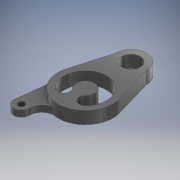
# Autodesk Inventor part: LR3_2
Saved by Autodesk Inventor 2018 (Build 220112000, 112)
## iProperties
Created: 2020-04-08
Part Number: LR3_2
Material: Типовые
Document SubType Name: Modeling
Designer: Siarhei
Density: 1 g/cm^3
Appearance: По умолчанию
Author: Siarhei
Autodesk Inventor part; units mm, degrees
ref_plane "YZ Plane" through (0, 0, 0) normal (1, 0, 0) x (0, 1, 0)
ref_plane "XZ Plane" through (0, 0, 0) normal (0, 1, 0) x (-1, 0, 0)
ref_plane "XY Plane" through (0, 0, 0) normal (0, 0, 1) x (1, 0, 0)
sketch "Эскиз1" plane through (0, 0, 0) normal (0, 0, 1) x (1, 0, 0)
  circle A0 centre (0, 0) radius 5
  circle A1 centre (0, 0) radius 12.5
  arc A2 (-2.4853, 79.8323) -> (82.4853, 79.8323) centre (40, 65) ccw
  arc A3 (57.6777, 47.3223) -> (22.3223, 47.3223) centre (40, 65) ccw construction
  arc A4 (64.7487, 40.2513) -> (15.2513, 40.2513) centre (40, 65) ccw
  arc A5 (50.6066, 54.3934) -> (29.3934, 54.3934) centre (40, 65) ccw
  arc A6 (50.6066, 54.3934) -> (64.7487, 40.2513) centre (57.6777, 47.3223) ccw
  arc A7 (15.2513, 40.2513) -> (29.3934, 54.3934) centre (22.3223, 47.3223) ccw
  line L0 (40, 65) -> (57.6777, 47.3223) construction
  line L1 (40, 65) -> (65, 65) construction
  line L2 (40, 65) -> (22.3223, 47.3223) construction
  line L3 (-12.5, 0) -> (-5, 65)
  circle A8 centre (40, 140) radius 15
  arc A9 (65, 140) -> (15, 140) centre (40, 140) ccw
  line L4 (15, 140) -> (-3.8175, 75.2482)
  line L5 (65, 140) -> (83.8175, 75.2482)
  arc A10 (31.1612, 20.8766) -> (12.5, 0) centre (32.4788, 0.92) ccw
  dimension "d0" = 10
  dimension "d1" = 25
  dimension "d2" = 90
  dimension "d4" = 25
  dimension "d5" = 45
  dimension "d6" = 90
  dimension "d7" = 20
  dimension "d9" = 30
  dimension "d10" = 50
  dimension "d11" = 20
  dimension "d24" = 73.796
  dimension "d25" = 32.409
  dimension "d26" = 22.786
  dimension "d27" = 101.4868
  dimension "d28" = 65
  dimension "d29" = 74.2462
  dimension "d30" = 24.665
  dimension "d31" = 12.4176
  dimension "d32" = 75
  dimension "d33" = 24.0068
  dimension "d34" = 70.0415
  dimension "d35" = 64.0799
  constraints: 22 point on circle, 12 end point, 11 centre point, 4 coincident, 4 tangent, 2 point on line, 1 equal length, 1 horizontal
  measures "d0" diameter of A0
  measures "d1" diameter of A1
  measures "d2" diameter of A2
  measures "d4" radius of A3
  measures "d5" angle of L0 L1
  measures "d6" angle of L2 L0
  measures "d7" diameter of A7
  measures "d9" diameter of A8
  measures "d10" diameter of A9
  measures "d11" radius of A10
  measures "d24" angle of L5 L1
  measures "d25" angle of L4 L5
  measures "d26" angle of L3 L5
  measures "d27" distance from line of point (0, 0) L5
  measures "d28" distance from line of point (0, 0) L1
  measures "d29" distance from line of point (0, 0) L0
  measures "d30" distance from line of point (0, 0) L4
  measures "d31" distance from line of point (0, 0) L3
  measures "d32" distance from line of L5.start L1
  measures "d33" distance from line of A9.centre L5
  measures "d34" distance from line of A10.centre L5
  measures "d35" distance from line of A10.centre L1
extrude "Выдавливание1" add sketch "Эскиз1" along normal blind 10 contours L3 A1 A10 | L3 A2 A10 A1
extrude "Выдавливание2" add sketch "Эскиз1" along normal blind 20 contours A2 L4 A9 L5
